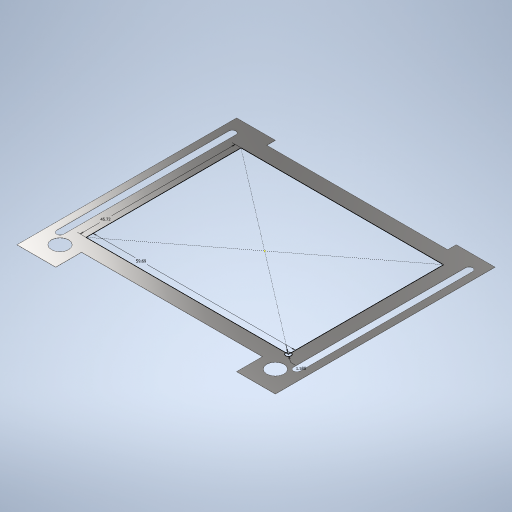
# Autodesk Inventor part: Module PCB Stencil - V1
Saved by Autodesk Inventor 2023 (Build 270158000, 158)
## iProperties
Created: 2022-06-23
Part Number: Module PCB Stencil - V1
Material: Stainless Steel
Document SubType Name: Modeling
Designer: Caleb
Density: 8 g/cm^3
Appearance: Semi-Polished
Author: Caleb
Autodesk Inventor part; units mm, degrees
ref_plane "YZ Plane" through (0, 0, 0) normal (1, 0, 0) x (0, 1, 0)
ref_plane "XZ Plane" through (0, 0, 0) normal (0, 1, 0) x (-1, 0, 0)
ref_plane "XY Plane" through (0, 0, 0) normal (0, 0, 1) x (1, 0, 0)
sketch "Sketch1" plane through (0, 0, 0) normal (0, 1, 0) x (-1, 0, 0)
  line L0 (-38.1, -34.925) -> (38.1, -34.925)
  line L1 (38.1, -34.925) -> (38.1, 34.925)
  line L2 (38.1, 34.925) -> (-38.1, 34.925)
  line L3 (-38.1, 34.925) -> (-38.1, -34.925)
  line L4 (-38.1, -34.925) -> (38.1, 34.925) construction
  line L5 (38.1, -34.925) -> (-38.1, 34.925) construction
  point P0 (0, 0)
  dimension "d0" = 76.2
  dimension "d1" = 69.85
  constraints: 12 end point, 2 midpoint, 2 parallel, 1 horizontal, 1 perpendicular
  measures "d0" distance of L2.end L1.end
  measures "d1" distance of L1.end L0.end
extrude "Extrusion1" add sketch "Sketch1" along normal blind 0.0508
sketch "Sketch2" plane through (0, 0.0508, 0) normal (0, 1, 0) x (1, 0, 0)
  line L0 (34.925, -25.4) -> (34.925, 25.4) construction
  line L1 (35.941, -25.4) -> (35.941, 25.4)
  line L2 (33.909, 25.4) -> (33.909, -25.4)
  arc A0 (33.909, -25.4) -> (35.941, -25.4) centre (34.925, -25.4) ccw
  arc A1 (35.941, 25.4) -> (33.909, 25.4) centre (34.925, 25.4) ccw
  line L3 (38.1, -34.925) -> (38.1, 34.925) projected
  line L4 (0, -11.2063) -> (0, 14.7333)
  line L5 (-34.925, -25.4) -> (-34.925, 25.4) construction
  line L6 (-35.941, -25.4) -> (-35.941, 25.4)
  line L7 (-33.909, 25.4) -> (-33.909, -25.4)
  arc A2 (-35.941, -25.4) -> (-33.909, -25.4) centre (-34.925, -25.4) ccw
  arc A3 (-33.909, 25.4) -> (-35.941, 25.4) centre (-34.925, 25.4) ccw
  line L8 (-38.1, -34.925) -> (38.1, -34.925) projected
  line L9 (-38.1, 34.925) -> (-38.1, -34.925) projected
  point P0 (0, 0)
  point P1 (34.925, 0)
  point P2 (-34.925, 0)
  point P3 (31.75, -28.575)
  point P4 (-31.75, -28.575)
  dimension "d4" = 2.032
  dimension "d5" = 3.175
  dimension "d6" = 50.8
  dimension "d14" = 6.35
  dimension "d15" = 6.35
  dimension "d16" = 6.35
  dimension "d17" = 6.35
  constraints: 18 end point, 8 point on circle, 7 symmetric about line, 4 centre point, 4 tangent, 2 vertical, 1 horizontal alignment, 1 midpoint, 1 parallel, 2 other
  measures "d4" distance between parallel lines of L2 L1
  measures "d5" distance from line of L3 point (34.925, 0)
  measures "d6" distance of L0.end L0.start
  measures "d14" distance from line of L3 point (31.75, -28.575)
  measures "d15" distance from line of L8 point (31.75, -28.575)
  measures "d16" distance from line of L8 point (-31.75, -28.575)
  measures "d17" distance from line of L9 point (-31.75, -28.575)
extrude "Extrusion2" cut sketch "Sketch2" against normal through all
sketch "Sketch3" plane through (0, 0.0508, 0) normal (0, 1, 0) x (1, 0, 0)
  line L0 (-38.1, -34.925) -> (38.1, -34.925) projected
  line L1 (-26.67, -34.925) -> (26.67, -34.925)
  line L2 (26.67, -34.925) -> (26.67, -27.305)
  line L3 (26.67, -27.305) -> (-26.67, -27.305)
  line L4 (-26.67, -27.305) -> (-26.67, -34.925)
  line L5 (-38.1, 34.925) -> (-38.1, -34.925) projected
  line L6 (15.3292, 0) -> (-25.2672, 0)
  line L7 (-26.67, 34.925) -> (26.67, 34.925)
  line L8 (26.67, 34.925) -> (26.67, 27.305)
  line L9 (26.67, 27.305) -> (-26.67, 27.305)
  line L10 (-26.67, 27.305) -> (-26.67, 34.925)
  point P0 (0, 0)
  dimension "d9" = 7.62
  dimension "d10" = 53.34
  dimension "d11" = 11.43
  constraints: 18 end point, 4 symmetric about line, 2 horizontal, 2 parallel, 1 perpendicular, 1 point on line
  measures "d9" distance of L3.end L1.start
  measures "d10" distance between parallel lines of L4 L2
  measures "d11" distance between parallel lines of L5 L4
extrude "Extrusion3" cut sketch "Sketch3" against normal through all
sketch "Sketch4" plane through (0, 0.0508, 0) normal (0, 1, 0) x (1, 0, 0)
  line L0 (-38.1, 34.925) -> (-38.1, -34.925) projected
  line L1 (-38.1, -34.925) -> (-26.67, -34.925) projected
  line L2 (26.67, -34.925) -> (38.1, -34.925) projected
  line L3 (38.1, -34.925) -> (38.1, 34.925) projected
  point P0 (0, 0)
  point P1 (-31.75, -28.575)
  point P2 (31.75, -28.575)
  dimension "d18" = 6.35
  dimension "d19" = 6.35
  dimension "d20" = 6.35
  dimension "d21" = 6.35
  measures "d18" distance from line of L0 point (-31.75, -28.575)
  measures "d19" distance from line of L1 point (-31.75, -28.575)
  measures "d20" distance from line of L2 point (31.75, -28.575)
  measures "d21" distance from line of point (31.75, -28.575) L3
hole "Hole1" at (-31.75, 0.0508, 28.575) at (31.75, 0.0508, 28.575) direction (0, -1, 0) diameter 5.08 end through all
sketch "Sketch5" plane through (0, 0.0508, 0) normal (0, 1, 0) x (1, 0, 0)
  line L0 (-26.67, 34.925) -> (-38.1, 34.925) projected
  line L1 (38.1, -34.925) -> (38.1, 34.925) projected
  line L2 (-38.1, 34.925) -> (38.1, 34.925)
  line L3 (38.1, 34.925) -> (38.1, 29.845)
  line L4 (38.1, 29.845) -> (-38.1, 29.845)
  line L5 (-38.1, 29.845) -> (-38.1, 34.925)
  point P0 (0, 0)
  dimension "d29" = 5.08
  constraints: 8 end point, 2 parallel, 1 horizontal, 1 perpendicular, 1 point on line
  measures "d29" distance between parallel lines of L4 L2
extrude "Extrusion4" cut sketch "Sketch5" against normal through all
sketch "Sketch6" plane through (0, 0.0508, 0) normal (0, 1, 0) x (1, 0, 0)
  line L0 (-29.845, 22.86) -> (29.845, 22.86)
  line L1 (29.845, 22.86) -> (29.845, -22.86)
  line L2 (29.845, -22.86) -> (-29.845, -22.86)
  line L3 (-29.845, -22.86) -> (-29.845, 22.86)
  line L4 (-29.845, 22.86) -> (29.845, -22.86) construction
  line L5 (29.845, 22.86) -> (-29.845, -22.86) construction
  circle A0 centre (29.845, -22.86) radius 0.7938
  point P0 (0, 0)
  point P1 (29.0512, -22.86)
  point P2 (29.845, -22.0662)
  dimension "d32" = 1.5875
  dimension "d33" = 45.72
  dimension "d34" = 59.69
  constraints: 12 end point, 2 midpoint, 2 parallel, 1 centre point, 1 coincident, 1 horizontal, 1 perpendicular
  measures "d32" diameter of A0
  measures "d33" distance of L2.end L0.start
  measures "d34" distance of L1.end L2.end
extrude "Extrusion5" cut sketch "Sketch6" against normal through all
equation "\"d15\" = d14"
equation "\"d16\" = d14"
equation "\"d17\" = d14"
equation "\"d19\" = d18"
equation "\"d20\" = d18"
equation "\"d21\" = d18"
body "Solid1"
